Autodesk Fusion 360 part; units mm, degrees
(part 2 of 2)
  circle A932 centre (301.2857, -8.2) radius 2.25
  circle A933 centre (310.7143, -8.2) radius 2.25
  circle A934 centre (320.1429, -8.2) radius 2.25
  circle A935 centre (329.5714, -8.2) radius 2.25
  circle A936 centre (339, -8.2) radius 2.25
  circle A937 centre (348.4286, -8.2) radius 2.25
  circle A938 centre (357.8571, -8.2) radius 2.25
  circle A939 centre (367.2857, -8.2) radius 2.25
  circle A940 centre (376.7143, -8.2) radius 2.25
  circle A941 centre (386.1429, -8.2) radius 2.25
  circle A942 centre (395.5714, -8.2) radius 2.25
  circle A943 centre (405, -8.2) radius 2.25
  dimension "d5" = 35
  dimension "d7" = 35
  dimension "d10" = 160
  dimension "d11" = 480
  dimension "d12" = 4.5
  dimension "d15" = 462
  dimension "d16" = 177.8
  constraint perpendicular L4 L5
  constraint perpendicular L1 L6
  constraint perpendicular L0 L7
  measures "d5" distance of L1.start L1.end
  measures "d7" distance of L3.start L3.end
  measures "d10" distance of L0.end L4.end
  measures "d11" distance of L0.start L0.end
  measures "d12" diameter of A0
extrude "Extrude1" add sketch "Sketch1" along normal blind 6.35
